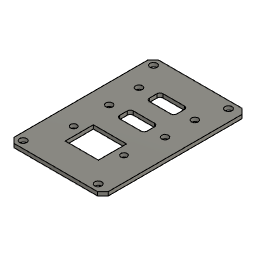
Side Panel - RJ-45 & Dual USB (Autodesk Fusion 360 design; units mm, degrees)
Autodesk Fusion 360 part; units mm, degrees
ref_plane "WorkPlane2" through (0, 0, 2.999) normal (0, 0, 1) x (1, 0, 0)
sketch "Sketch4" plane through (0, 0, 2.999) normal (0, 0, 1) x (1, 0, 0)
  line L0 (92.5002, -5.0854) -> (92.4954, -5.0854)
  line L1 (89.5002, -5.0854) -> (44.5002, -5.0854) construction
  line L2 (44.5002, -5.0854) -> (41.5002, -8.0854) construction
  line L3 (41.5002, -8.0854) -> (41.5002, -80.0854) construction
  line L4 (41.5002, -80.0854) -> (44.5002, -83.0854) construction
  line L5 (44.5002, -83.0854) -> (89.5002, -83.0854) construction
  line L6 (92.5002, -80.0854) -> (92.5002, -8.0854) construction
  line L7 (86.0002, -79.0854) -> (86.0002, -83.0854) construction
  line L8 (86.0002, -79.0854) -> (92.5002, -79.0854) construction
  line L9 (86.0002, -79.0854) -> (45.705, -79.088) construction
  line L10 (45.7002, -79.0828) -> (41.5002, -79.0831) construction
  line L11 (45.7002, -9.088) -> (45.7002, -5.0854) construction
  line L12 (45.7002, -9.088) -> (45.705, -79.088) construction
  line L13 (45.6956, -9.088) -> (85.9956, -9.0854) construction
  line L14 (85.9956, -9.0854) -> (92.5002, -9.0854) construction
  line L15 (85.9956, -9.0854) -> (85.9956, -5.0854) construction
  line L16 (85.9956, -79.0854) -> (85.9931, -9.0854) construction
  line L17 (92.5002, -80.0854) -> (89.5002, -83.0854) construction
  line L18 (92.5002, -8.0854) -> (89.5002, -5.0854) construction
  line L19 (44.583, -82.8854) -> (89.4174, -82.8854)
  line L20 (92.3002, -80.0026) -> (89.4174, -82.8854)
  line L21 (92.3002, -80.0026) -> (92.3002, -8.1683)
  line L22 (92.3002, -8.1683) -> (89.4174, -5.2854)
  line L23 (89.4174, -5.2854) -> (44.583, -5.2854)
  line L24 (44.583, -5.2854) -> (41.7002, -8.1683)
  line L25 (41.7002, -8.1683) -> (41.7002, -80.0026)
  line L26 (41.7002, -80.0026) -> (44.583, -82.8854)
  circle A0 centre (85.9956, -9.0854) radius 1.9
  circle A1 centre (45.7002, -9.088) radius 1.9
  circle A2 centre (85.9956, -79.0854) radius 1.9
  circle A3 centre (45.7002, -79.0828) radius 1.9
  line L27 (92.5002, -44.0854) -> (41.5002, -44.0854) construction
  point P0 (92.5002, -83.0854)
  point P1 (92.5002, -5.0854)
  dimension "d34" = 6.5
  dimension "d35" = 4
  dimension "d36" = 4.2
  dimension "d37" = 40.2952
  dimension "d38" = 4
  dimension "d39" = 3
  dimension "d40" = 3
  dimension "d43" = 78
  dimension "d44" = 3
  dimension "d45" = 3
  dimension "d46" = 3
  dimension "d47" = 3
  dimension "d48" = 3
  dimension "d49" = 3
  dimension "d50" = -0.2
  dimension "d53" = 3.8
  dimension "d54" = 3.8
  dimension "d55" = 3.8
  dimension "d56" = 3.8
  dimension "d57" = 51
  constraint coincident L5 L7.end
  constraint perpendicular L5 L7
  constraint coincident L6 L8.end
  constraint perpendicular L6 L8
  constraint coincident L3 L10.end
  constraint coincident L1 L11.end
  constraint perpendicular L1 L11
  constraint perpendicular L10 L12
  constraint coincident L6 L14.end
  constraint perpendicular L6 L14
  constraint coincident L1 L15.end
  constraint perpendicular L1 L15
  constraint horizontal L1
  constraint vertical L6
  constraint horizontal L5
  constraint vertical L3
  constraint coincident P0 L6
  constraint coincident P0 L5
  constraint coincident L6 P1
  constraint coincident L1 P1
  constraint coincident L0.start L6
  constraint coincident L0.end L1
  constraint coincident L13.end L14.start
  constraint coincident L11.start L12.start
  constraint coincident L16.start A2.centre
  constraint coincident L10.start A3.centre
  constraint midpoint L6 L27.start
  constraint midpoint L3 L27.end
  constraint symmetric A1 A3 L27
  constraint symmetric A0 A2 L27
  measures "d34" horizontal distance of L7.start L8.end
  measures "d35" vertical distance of L7.start L7.end
  measures "d36" horizontal distance of L10.start L10.end
  measures "d37" horizontal distance of L7.start L9.end
  measures "d38" vertical distance of L13.end L15.end
  measures "d39" horizontal distance of L1.end L2.end
  measures "d40" vertical distance of L1.end L2.end
  measures "d43" distance of L1 L5
  measures "d44" horizontal distance of L3.end L4.end
  measures "d45" vertical distance of L3.end L4.end
  measures "d46" distance of P0 L6.start
  measures "d47" distance of P0 L5.end
  measures "d48" distance of L6.end P1
  measures "d49" distance of L1.start P1
  measures "d53" diameter of A0
  measures "d54" diameter of A1
  measures "d55" diameter of A2
  measures "d56" diameter of A3
  measures "d57" distance of L3 L6
extrude "Extrude11" add sketch "Sketch4" against normal blind 2
sketch "Sketch5" plane through (0, 0, 2.999) normal (0, 0, 1) x (-1, 0, 0)
  circle A0 centre (-85.9956, 9.0854) radius 1.9
  circle A1 centre (-45.7002, 79.0828) radius 1.9
  circle A2 centre (-85.9956, 79.0854) radius 1.9
  circle A3 centre (-45.7002, 9.088) radius 1.9
  line L0 (-92.3002, 80.0026) -> (-92.3002, 8.1683)
  line L1 (-92.3002, 8.1683) -> (-89.4174, 5.2854)
  line L2 (-89.4174, 5.2854) -> (-44.583, 5.2854)
  line L3 (-44.583, 5.2854) -> (-41.7002, 8.1683)
  line L4 (-41.7002, 8.1683) -> (-41.7002, 80.0026)
  line L5 (-41.7002, 80.0026) -> (-44.583, 82.8854)
  line L6 (-44.583, 82.8854) -> (-89.4174, 82.8854)
  line L7 (-89.4174, 82.8854) -> (-92.3002, 80.0026)
  arc A4 (-74.5502, 21.3354) -> (-72.9502, 19.7354) centre (-72.9502, 21.3354) ccw
  line L8 (-67.2002, 23.3854) -> (-52.2002, 23.3854) construction
  line L9 (-87.2002, 30.8854) -> (-87.2002, 15.8854)
  line L10 (-87.2002, 15.8854) -> (-47.2002, 30.8854) construction
  line L11 (-72.9502, 19.7354) -> (-61.4502, 19.7354)
  arc A5 (-59.8502, 25.4354) -> (-61.4502, 27.0354) centre (-61.4502, 25.4354) ccw
  line L12 (-61.4502, 27.0354) -> (-72.9502, 27.0354)
  line L13 (-74.5502, 19.7354) -> (-59.8502, 27.0354) construction
  circle A6 centre (-52.2002, 23.3854) radius 1.8
  arc A7 (-72.9502, 27.0354) -> (-74.5502, 25.4354) centre (-72.9502, 25.4354) ccw
  line L14 (-87.2002, 15.8854) -> (-47.2002, 15.8854)
  line L15 (-47.2002, 30.8854) -> (-87.2002, 30.8854)
  circle A8 centre (-82.2002, 23.3854) radius 1.8
  line L16 (-74.5502, 25.4354) -> (-74.5502, 21.3354)
  line L17 (-47.2002, 15.8854) -> (-87.2002, 30.8854) construction
  line L18 (-59.8502, 19.7354) -> (-74.5502, 27.0354) construction
  line L19 (-59.8502, 21.3354) -> (-59.8502, 25.4354)
  line L20 (-47.2002, 15.8854) -> (-47.2002, 30.8854)
  arc A9 (-61.4502, 19.7354) -> (-59.8502, 21.3354) centre (-61.4502, 21.3354) ccw
  line L21 (-67.2002, 30.8854) -> (-67.2002, 23.3854) construction
  line L22 (-47.2002, 46.8854) -> (-87.2002, 46.8854)
  line L23 (-87.2002, 46.8854) -> (-87.2002, 31.8854)
  line L24 (-87.2002, 31.8854) -> (-47.2002, 31.8854)
  line L25 (-47.2002, 31.8854) -> (-47.2002, 46.8854)
  line L26 (-59.8502, 37.3354) -> (-59.8502, 41.4354)
  arc A10 (-59.8502, 41.4354) -> (-61.4502, 43.0354) centre (-61.4502, 41.4354) ccw
  line L27 (-61.4502, 43.0354) -> (-72.9502, 43.0354)
  arc A11 (-72.9502, 43.0354) -> (-74.5502, 41.4354) centre (-72.9502, 41.4354) ccw
  line L28 (-74.5502, 41.4354) -> (-74.5502, 37.3354)
  arc A12 (-74.5502, 37.3354) -> (-72.9502, 35.7354) centre (-72.9502, 37.3354) ccw
  arc A13 (-61.4502, 35.7354) -> (-59.8502, 37.3354) centre (-61.4502, 37.3354) ccw
  line L29 (-72.9502, 35.7354) -> (-61.4502, 35.7354)
  circle A14 centre (-52.2002, 39.3854) radius 1.8
  circle A15 centre (-82.2002, 39.3854) radius 1.8
  line L30 (-75, 52.9) -> (-75, 68)
  line L31 (-66.1, 60.45) -> (-66.1, 58.85) construction
  line L32 (-57.2, 52.9) -> (-75, 68) construction
  line L33 (-75, 52.9) -> (-57.2, 68) construction
  line L34 (-57.2, 52.9) -> (-75, 52.9)
  line L35 (-75, 68) -> (-57.2, 68)
  line L36 (-48.6, 72.95) -> (-83.6, 47.95) construction
  line L37 (-48.6, 47.95) -> (-48.6, 72.95)
  line L38 (-57.2, 68) -> (-57.2, 52.9)
  circle A16 centre (-52.6, 58.85) radius 1.675
  line L39 (-79.6, 58.85) -> (-52.6, 58.85) construction
  line L40 (-83.6, 72.95) -> (-48.6, 47.95) construction
  line L41 (-48.6, 72.95) -> (-83.6, 72.95)
  circle A17 centre (-79.6, 58.85) radius 1.675
  line L42 (-83.6, 72.95) -> (-83.6, 47.95)
  line L43 (-83.6, 47.95) -> (-48.6, 47.95)
  line L44 (-66.1, 60.45) -> (-61, 60.45) construction
  point P0 (-67.2002, 25.3854)
  point P1 (-67.2002, 23.3854)
  point P2 (-75, 68)
  point P3 (-66.1, 60.45)
  dimension "d555" = 14.7
  dimension "d556" = 7.3
  dimension "d557" = 1.6
  dimension "d558" = 1.6
  dimension "d559" = 1.6
  dimension "d560" = 1.6
  dimension "d561" = 15
  dimension "d562" = 3.6
  dimension "d240" = 15
  dimension "d241" = 40
  dimension "d68" = 1.6
  dimension "d69" = 1.6
  dimension "d70" = 1.6
  dimension "d71" = 1.6
  dimension "d72" = 3.6
  dimension "d73" = 15
  dimension "d74" = 40
  dimension "d596" = 3.35
  dimension "d597" = 3.35
  dimension "d244" = 1.6
  dimension "d245" = 15.1
  dimension "d246" = 17.8
  dimension "d247" = 27
  dimension "d248" = 35
  dimension "d249" = 25
  constraint perpendicular L11 L19
  constraint parallel L11 L12
  constraint parallel L16 L19
  constraint coincident L18.start L11
  constraint coincident L18.start L19
  constraint tangent L11 A9
  constraint tangent L19 A9
  constraint coincident L13.start L16
  constraint coincident L13.start L11
  constraint tangent A4 L16
  constraint tangent A4 L11
  constraint coincident L18.end L16
  constraint coincident L18.end L12
  constraint tangent A7 L16
  constraint tangent L12 A7
  constraint coincident L13.end L19
  constraint coincident L13.end L12
  constraint tangent A5 L19
  constraint tangent A5 L12
  constraint perpendicular L8 L19
  constraint coincident L8.end A6.centre
  constraint perpendicular L14 L20
  constraint parallel L14 L15
  constraint parallel L9 L20
  constraint coincident P1 L10
  constraint coincident P1 L17
  constraint coincident P1 L8.start
  constraint midpoint L21.start L15
  constraint symmetric A6 A8 L21
  constraint perpendicular L26 L29
  constraint parallel L27 L29
  constraint parallel L26 L28
  constraint tangent A13 L29
  constraint tangent L26 A13
  constraint tangent L28 A12
  constraint tangent A12 L29
  constraint tangent A11 L28
  constraint tangent L27 A11
  constraint tangent L26 A10
  constraint tangent A10 L27
  constraint perpendicular L24 L25
  constraint parallel L22 L24
  constraint parallel L23 L25
  constraint coincident L39.start A17.centre
  constraint coincident A16.centre L39.end
  constraint perpendicular L38 L39
  constraint midpoint P3 L32
  constraint midpoint L31.end L39
  constraint horizontal L41
  constraint perpendicular L41 L42
  constraint parallel L41 L43
  constraint parallel L37 L42
  constraint coincident P3 L36
  constraint coincident P3 L40
  constraint coincident P3 L31.start
  constraint perpendicular L31 L44
  constraint symmetric L41 L43 L44
  measures "d555" distance of L18.end L13.end
  measures "d556" distance of L18.start L13.end
  measures "d557" radius of A9
  measures "d558" radius of A4
  measures "d559" radius of A7
  measures "d560" radius of A5
  measures "d561" distance of L8.end P1
  measures "d562" diameter of A6
  measures "d240" distance of L14.end L10.end
  measures "d241" distance of L9.start L10.end
  measures "d68" radius of A13
  measures "d69" radius of A12
  measures "d70" radius of A11
  measures "d71" radius of A10
  measures "d72" diameter of A14
  measures "d73" distance of L22.start L24.end
  measures "d74" distance of L22.start L22.end
  measures "d596" diameter of A17
  measures "d597" diameter of A16
  measures "d244" distance of L31.end P3
  measures "d245" distance of P2 L30.start
  measures "d246" distance of L32.start L30.start
  measures "d247" distance of A16.centre L39.start
  measures "d248" distance of L36.end L37.start
  measures "d249" distance of L40.start L36.end
extrude "Extrude12" cut sketch "Sketch5" against normal blind 2 contours A4 L11 A5 L12 A7 L16 L19 A9 | A6 | A8 | L26 A10 L27 A11 L28 A12 A13 L29 | A14 | A15 | L30 L34 L35 L38 | A16 | A17
equation "d39 = d40"
equation "d40 = d44"
equation "d45 = d44"
equation "d46 = d44"
equation "d47 = d46"
equation "d48 = d44"
equation "d49 = d48"
equation "d53 = d55"
equation "d54 = d55"
equation "d56 = d55"
equation "d558 = d557"
equation "d559 = d557"
equation "d560 = d557"
equation "d69 = d557"
equation "d70 = d557"
equation "d71 = d557"
equation "d596 = M3_hole_dia_Ref"
equation "d597 = M3_hole_dia_Ref"
